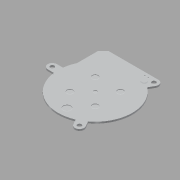
# Autodesk Inventor part: PCB
Saved by Autodesk Inventor 2020 (Build 240168000, 168)
## iProperties
Created: 2020-07-09
Part Number: PCB
Material: Generic
Document SubType Name: Modeling
Designer: user
Density: 1 g/cm^3
Appearance: Smooth - Dark Forest Green
Author: user
Autodesk Inventor part; units mm, degrees
ref_plane "YZ Plane" through (0, 0, 0) normal (1, 0, 0) x (0, 1, 0)
ref_plane "XZ Plane" through (0, 0, 0) normal (0, 1, 0) x (-1, 0, 0)
ref_plane "XY Plane" through (0, 0, 0) normal (0, 0, 1) x (1, 0, 0)
sketch "Sketch1" plane through (0, 0, 0) normal (0, 1, 0) x (-1, 0, 0)
  circle A0 centre (42.5, 0) radius 2
  circle A1 centre (-21.25, 36.8061) radius 2
  circle A2 centre (-21.25, -36.8061) radius 2
  line L0 (-21.25, -36.8061) -> (0, 0) construction
  arc A3 (-25.1562, -34.5508) -> (-20.8492, -41.2987) centre (-21.25, -36.8061) ccw
  line L1 (-21.25, 36.8061) -> (0, 0) construction
  arc A4 (-17.3438, 39.0613) -> (-25.1562, 34.5508) centre (-21.25, 36.8061) ccw
  line L2 (0, 0) -> (42.5, 0) construction
  arc A5 (42.5, -4.5105) -> (42.5, 4.5105) centre (42.5, 0) ccw
  line L3 (-21.6508, -41.2987) -> (28.2014, -41.2987)
  line L4 (28.2014, -41.2987) -> (33.3458, -35.9407)
  line L5 (33.3458, -35.9407) -> (33.3458, -15.3261)
  line L6 (-25.1562, -34.5508) -> (-22.1167, -29.2863)
  line L7 (36.421, -4.5105) -> (42.5, -4.5105)
  line L8 (42.5, 0) -> (36.6992, 0)
  line L9 (4.5105, 0) -> (0, 0)
  line L10 (42.5, 4.5105) -> (36.421, 4.5105)
  line L11 (-25.1562, 34.5508) -> (-22.1167, 29.2863)
  line L12 (-14.3043, 33.7968) -> (-17.3438, 39.0613)
  arc A6 (-22.1167, 29.2863) -> (-22.1167, -29.2863) centre (0, 0) ccw
  arc A7 (33.3458, -15.3261) -> (36.421, -4.5105) centre (0, 0) ccw
  arc A8 (36.421, 4.5105) -> (-14.3043, 33.7968) centre (0, 0) ccw
  point P0 (-10.625, -18.403)
  point P1 (-10.625, 18.403)
  point P2 (21.25, 0)
  dimension "d1" = 4
  dimension "d2" = 42.5
  dimension "d5" = 360
  constraints: 32 end point, 13 point on circle, 9 centre point, 5 tangent, 4 horizontal, 3 midpoint, 2 coincident, 2 parallel, 1 perpendicular, 1 point on line, 7 other
  measures "d1" diameter of A0
  measures "d2" distance of L2.end L9.end
extrude "Extrusion1" add sketch "Sketch1" along normal blind 1.6 contours L6 A6 L11 A4 L12 A8 L10 A5 L7 A7 L5 L4 L3 A3
sketch "Sketch2" plane through (0, 1.6, 0) normal (0, 1, 0) x (1, 0, 0)
  line L0 (35, 0) -> (0, 0) construction
  circle A0 centre (12.5, 12.5) radius 3
  circle A1 centre (-12.5, 12.5) radius 3
  circle A2 centre (-12.5, -12.5) radius 3
  circle A3 centre (12.5, -12.5) radius 3
  line L1 (1.675, -1.675) -> (-1.675, -1.675)
  line L2 (-1.675, -1.675) -> (-1.675, 1.675)
  line L3 (-1.675, 1.675) -> (1.675, 1.675)
  line L4 (1.675, 1.675) -> (1.675, -1.675)
  line L5 (1.675, -1.675) -> (-1.675, 1.675) construction
  line L6 (-1.675, -1.675) -> (1.675, 1.675) construction
  circle A4 centre (0, 0) radius 1.675
  circle A5 centre (0, -28) radius 3.75
  line L7 (0, -28) -> (0, 0) construction
  line L8 (-42.5, -4.5105) -> (-36.421, -4.5105) projected
  arc A6 (-42.5, 4.5105) -> (-42.5, -4.5105) centre (-42.5, 0) ccw projected
  line L9 (-36.421, 4.5105) -> (-42.5, 4.5105) projected
  arc A7 (-33.3458, 15.3261) -> (-36.421, 4.5105) centre (0, 0) ccw projected
  line L10 (-33.3458, 35.9407) -> (-33.3458, 15.3261) projected
  line L11 (-28.2014, 41.2987) -> (-33.3458, 35.9407) projected
  line L12 (21.6508, 41.2987) -> (-28.2014, 41.2987) projected
  arc A8 (25.1562, 34.5508) -> (21.6508, 41.2987) centre (21.25, 36.8061) ccw projected
  line L13 (22.1167, 29.2863) -> (25.1562, 34.5508) projected
  arc A9 (22.1167, -29.2863) -> (22.1167, 29.2863) centre (0, 0) ccw projected
  line L14 (25.1562, -34.5508) -> (22.1167, -29.2863) projected
  arc A10 (17.3438, -39.0613) -> (25.1562, -34.5508) centre (21.25, -36.8061) ccw projected
  line L15 (14.3043, -33.7968) -> (17.3438, -39.0613) projected
  arc A11 (-36.421, -4.5105) -> (14.3043, -33.7968) centre (0, 0) ccw projected
  circle A12 centre (21.25, 36.8061) radius 2 projected
  circle A13 centre (21.25, -36.8061) radius 2 projected
  circle A14 centre (-42.5, 0) radius 2 projected
  circle A15 centre (11, 38.1) radius 0.381
  circle A16 centre (14.4, 38.1) radius 0.381
  line L16 (11, 38.1) -> (14.4, 38.1) construction
  dimension "d23" = 35
  dimension "d24" = 360
  dimension "d25" = 12.5
  dimension "d26" = 12.5
  dimension "d27" = 6
  dimension "d28" = 360
  dimension "d31" = 3.35
  dimension "d32" = 28
  dimension "d33" = 7.5
  dimension "d34" = 11
  dimension "d36" = 38.1
  dimension "d37" = 3.4
  dimension "d38" = 0.762
  constraints: 18 end point, 8 centre point, 3 coincident, 3 horizontal, 3 perpendicular, 2 midpoint, 2 parallel, 1 equal radius, 9 other
  measures "d23" distance of L0.start L0.end
  measures "d25" horizontal distance of point (0, 0) A0.centre
  measures "d26" horizontal distance of A0.centre point (0, 0)
  measures "d27" diameter of A0
  measures "d31" distance of L1.end L2.end
  measures "d32" distance of point (0, 0) L7.start
  measures "d33" diameter of A5
  measures "d34" horizontal distance of point (0, 0) L16.start
  measures "d36" distance from line of point (0, 0) L16
  measures "d37" distance of L16.start L16.end
  measures "d38" diameter of A16
extrude "Extrusion2" cut sketch "Sketch2" against normal blind 0.5 contours A0 | A1 | A2 | A3 | A4 | A5 | A15 | A16
sketch "Sketch3" plane through (0, 0, 0) normal (0, -1, 0) x (1, 0, 0)
  line L0 (14.38, -37.6973) -> (11.88, -37.6973)
  line L1 (21.6508, -41.2987) -> (-28.2014, -41.2987) construction
  line L2 (11.88, -32.9109) -> (14.38, -32.9109)
  arc A0 (14.38, -37.6973) -> (14.38, -32.9109) centre (13.13, -35.3041) ccw
  arc A1 (11.88, -32.9109) -> (11.88, -37.6973) centre (13.13, -35.3041) ccw
  line L3 (11.88, -37.6973) -> (14.38, -32.9109) construction
  line L4 (14.38, -37.6973) -> (11.88, -32.9109) construction
  line L5 (14.4, -35.3041) -> (11.86, -35.3041) construction
  circle A2 centre (14.4, -35.3041) radius 0.381
  circle A3 centre (11.86, -35.3041) radius 0.381
  circle A4 centre (21.25, -36.8061) radius 2 construction
  point P0 (0, 0)
  dimension "d39" = 2.7
  dimension "d40" = 2.5
  dimension "d41" = 0.762
  dimension "d42" = 2.54
  dimension "d43" = 6.85
  dimension "d44" = 1.502
  constraints: 10 end point, 5 midpoint, 4 centre point, 4 point on circle, 2 coincident, 2 equal radius, 2 horizontal, 1 parallel
  measures "d39" radius of A1
  measures "d40" distance of L0.start L0.end
  measures "d41" diameter of A3
  measures "d42" distance of L5.start L5.end
  measures "d43" horizontal distance of L5.start A4.centre
  measures "d44" vertical distance of A4.centre L5.start
extrude "Extrusion3" add sketch "Sketch3" along normal blind 1 contours L0 A1 L2 A0 | A2 | A3
equation "\"d26\" = d25"
body "Solid1"
